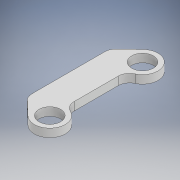
# Autodesk Inventor part: TelescopeMountConnector
Saved by Autodesk Inventor 2022 (Build 260153000, 153)
## iProperties
Created: 2021-05-06
Part Number: TelescopeMountConnector
Material: Generic
Document SubType Name: Modeling
Designer: Mick Veldhuis
Density: 1 g/cm^3
Appearance: Default
Author: Mick Veldhuis
Autodesk Inventor part; units mm, degrees
ref_plane "YZ Plane" through (0, 0, 0) normal (1, 0, 0) x (0, 1, 0)
ref_plane "XZ Plane" through (0, 0, 0) normal (0, 1, 0) x (-1, 0, 0)
ref_plane "XY Plane" through (0, 0, 0) normal (0, 0, 1) x (1, 0, 0)
sketch "Sketch1" plane through (0, 0, 0) normal (0, 1, 0) x (-1, 0, 0)
  arc A0 (0, 30) -> (20.6897, -21.7241) centre (0, 0) ccw
  arc A1 (20.6897, 201.7241) -> (0, 150) centre (0, 180) ccw
  line L0 (54, 10) -> (54, 170)
  line L1 (0, 150) -> (0, 30)
  line L2 (54, 10) -> (20.6897, -21.7241)
  line L3 (54, 170) -> (20.6897, 201.7241)
  constraints: 8 end point, 4 point on circle, 3 coincident, 2 centre point, 2 tangent, 2 vertical
extrude "Extrusion2" add sketch "Sketch1" along normal blind 16
hole "Hole3" at (0, 0, 180) at (0, 0, 0) direction (0, 1, 0) diameter 42 depth 16
fillet "Fillet3" radius 22 2 edges at (0, 8, 30) (0, 8, 150)
sketch "Sketch4" plane through (-54, 0, 10) normal (-1, 0, 0) x (0, 0, 1)
  line L0 (0, 0) -> (0, 16) projected
  line L1 (0, 8) -> (160, 8)
  line L2 (160, 0) -> (160, 16) projected
  point P0 (-10, 0)
  point P1 (20, 8)
  point P2 (140, 8)
  constraints: 2 end point, 2 midpoint, 2 point on line
fillet "Fillet4" radius 22 2 edges at (-54, 8, 10) (-54, 8, 170)
hole "Hole4" at (-54, 8, 30) at (-54, 8, 150) direction (1, 0, 0) diameter 6.647 depth 20 tip angle 118 thread size "M8x1.25" class "6H" standard "ISO Metric profile"
body "Solid2"
